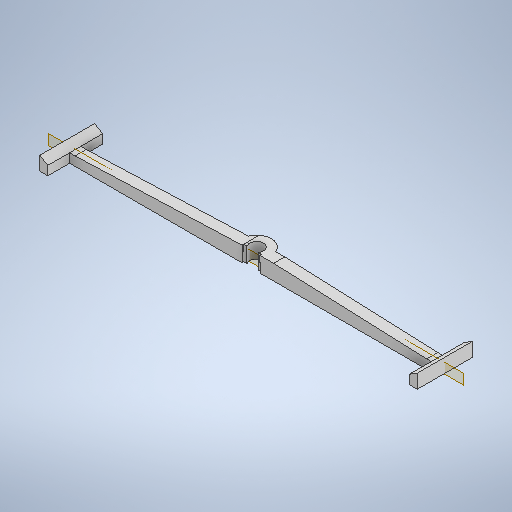
# Autodesk Inventor part: 2024_08_23_Holder_NMR_tube
Saved by Autodesk Inventor 2025.1 (Build 291241000, 241)
## iProperties
Created: 2024-08-23
Part Number: 2024_08_23_Holder_NMR_tube
Material: Generisch
Document SubType Name: Modeling
Designer: to86hug
Density: 1 g/cm^3
Appearance: Vorgabe
Author: to86hug
Autodesk Inventor part; units mm, degrees
ref_plane "YZ Plane" through (0, 0, 0) normal (1, 0, 0) x (0, 1, 0)
ref_plane "XZ Plane" through (0, 0, 0) normal (0, 1, 0) x (-1, 0, 0)
ref_plane "XY Plane" through (0, 0, 0) normal (0, 0, 1) x (1, 0, 0)
sketch "Skizze1" plane through (0, 0, 0) normal (0, 0, 1) x (1, 0, 0)
  line L0 (-68.016, 1.808) -> (67.584, 1.808)
  line L1 (67.584, 1.808) -> (67.584, -2.192)
  line L2 (67.584, -2.192) -> (-68.016, -2.192)
  line L3 (-68.016, -2.192) -> (-68.016, 1.808)
  line L4 (-68.016, 1.808) -> (67.584, -2.192) construction
  line L5 (67.584, 1.808) -> (-68.016, -2.192) construction
  point P0 (0, 0)
  point P1 (-0.216, -0.192)
  point P2 (-0.216, -0.192)
  dimension "d0" = 135.6
  dimension "d1" = 4
  constraints: 12 end point, 2 midpoint, 2 parallel, 1 horizontal, 1 perpendicular
  measures "d0" distance of L0.start L0.end
  measures "d1" distance of L0.end L1.end
extrude "Extrusion1" add sketch "Skizze1" along normal mid plane 3.25
ref_plane "Arbeitsebene1" through (-68.016, -0.192, 1.625) normal (0, -1, 0) x (1, 0, 0)
sketch "Skizze2" plane through (-68.016, -0.192, 1.625) normal (0, -1, 0) x (1, 0, 0)
  line L0 (0, -3.25) -> (0, 0) projected
  line L1 (0, -3.25) -> (135.6, -3.25) projected
  line L2 (0, 0) -> (2.85, 0)
  line L3 (2.85, 0) -> (2.85, -3.25)
  line L4 (2.85, -3.25) -> (0, -3.25)
  line L5 (0, -3.25) -> (0, 0)
  line L6 (0, 0) -> (0, 1.75)
  line L7 (0, 1.75) -> (2.85, 0)
  line L8 (135.6, -3.25) -> (135.6, 0) projected
  line L9 (135.6, 0) -> (132.75, 0)
  line L10 (132.75, 0) -> (132.75, -3.25)
  line L11 (132.75, -3.25) -> (135.6, -3.25)
  line L12 (135.6, -3.25) -> (135.6, 0)
  line L13 (135.6, 0) -> (135.6, 1.75)
  line L14 (135.6, 1.75) -> (132.75, 0)
  point P0 (68.016, -1.625)
  dimension "d4" = 2.85
  dimension "d5" = 1.75
  dimension "d6" = 2.85
  constraints: 24 end point, 4 parallel, 2 horizontal, 2 perpendicular, 2 point on line, 2 vertical
  measures "d4" distance of L3.end L4.end
  measures "d5" distance of L0.end L6.end
  measures "d6" distance of L11.end L10.end
extrude "Extrusion2" add sketch "Skizze2" along normal mid plane 19.7
sketch "Skizze3" plane through (0, 0, 1.625) normal (0, 0, 1) x (1, 0, 0)
  circle A0 centre (0, 0) radius 3.8975
  dimension "d9" = 7.795
  constraints: 1 centre point, 1 coincident
  measures "d9" diameter of A0
extrude "Extrusion3" cut sketch "Skizze3" against normal through all
sketch "Skizze4" plane through (0, 0, -1.625) normal (0, 0, -1) x (-1, 0, 0)
  line L0 (0.0769, -0.1614) -> (6.2269, -0.1614) construction
  circle A0 centre (0.0001, -0.1921) radius 2.495
  circle A1 centre (0.0001, -0.1921) radius 5.295
  line L1 (-24.5999, -1.5921) -> (24.6001, -1.5921)
  point P0 (-5.2949, -0.1921)
  point P1 (5.2951, -0.1921)
  point P2 (2.0653, -1.5921)
  point P3 (5.1066, -1.5921)
  point P4 (-5.1065, -1.5921)
  point P5 (-2.0651, -1.5921)
  dimension "d27" = 2.8
  dimension "d28" = 4.99
  dimension "d29" = 1.4
  constraints: 4 end point, 2 centre point, 2 coincident, 2 point on circle
  measures "d27" radial gap between concentric circles of A1 A0
  measures "d28" diameter of A0
  measures "d29" distance from line of A0.centre L1
extrude "Extrusion4" add sketch "Skizze4" against normal blind 5.5 contours A0 L1 A1 picked at (4.3097, 0.2335)
sketch "Skizze5" plane through (0, 0, 1.625) normal (0, 0, 1) x (1, 0, 0)
  line L0 (-4.9028, 1.808) -> (-65.166, 1.808) projected
  line L1 (-3.2227, -2.192) -> (-65.166, -2.192) projected
  line L2 (-3.2094, 1.808) -> (-63.2094, 1.808)
  line L3 (-63.2094, 1.808) -> (-63.2094, -2.192)
  line L4 (-63.2094, -2.192) -> (-3.2094, -2.192)
  line L5 (-3.2094, -2.192) -> (-3.2094, 1.808)
  line L6 (3.2227, -2.192) -> (64.734, -2.192) projected
  line L7 (3.1164, 1.808) -> (63.1164, 1.808)
  line L8 (63.1164, 1.808) -> (63.1164, -2.192)
  line L9 (63.1164, -2.192) -> (3.1164, -2.192)
  line L10 (3.1164, -2.192) -> (3.1164, 1.808)
  point P0 (0, 0)
  point P1 (-8.6889, 1.808)
  point P2 (-8.6001, -2.192)
  point P3 (8.6889, 1.808)
  point P4 (8.6001, -2.192)
  point P5 (3.1164, -2.192)
  point P6 (-3.2094, -2.192)
  point P7 (-63.2094, 1.808)
  point P8 (63.1164, -2.192)
  point P9 (-2.0688, 1.808)
  dimension "d17" = 60
  dimension "d18" = 60
  constraints: 16 end point, 4 parallel, 2 horizontal, 2 perpendicular
  measures "d17" distance of L4.end L3.end
  measures "d18" distance of L8.end L9.end
extrude "Extrusion5" add sketch "Skizze5" along normal blind 2.25
sketch "Skizze6" plane through (-65.166, -2.192, -1.625) normal (0, -1, 0) x (1, 0, 0)
  line L0 (1.9566, 5.5) -> (61.9566, 5.5) projected
  line L1 (1.9566, 5.5) -> (61.9566, 5.5)
  line L2 (56.9566, 5.5) -> (56.9566, 3.25)
  line L3 (56.9566, 3.25) -> (1.9566, 3.25)
  line L4 (1.9566, 3.25) -> (1.9566, 5.5)
  line L5 (61.9566, 5.5) -> (1.9566, 3.25)
  line L6 (128.2824, 3.25) -> (128.2824, 5.5) projected
  line L7 (128.2824, 5.5) -> (73.2824, 5.5)
  line L8 (73.2824, 5.5) -> (73.2824, 3.25)
  line L9 (73.2824, 3.25) -> (128.2824, 3.25)
  line L10 (128.2824, 3.25) -> (128.2824, 5.5)
  line L11 (73.2824, 5.5) -> (128.2824, 3.25)
  point P0 (65.166, 1.625)
  point P1 (56.5659, 5.5)
  point P2 (56.5659, 5.5)
  point P3 (56.5659, 5.5)
  dimension "d21" = 55
  dimension "d22" = 2.25
  dimension "d23" = 55
  dimension "d26" = 2.25
  constraints: 20 end point, 4 parallel, 2 horizontal, 2 perpendicular
  measures "d21" distance of L2.end L3.end
  measures "d22" vertical distance of L0.end L2.end
  measures "d23" distance of L9.end L8.end
  measures "d26" distance of L7.end L8.end
extrude "Extrusion6" cut sketch "Skizze6" against normal through all contours L0 L2 L5 L4 | L0 L5 L2 | L11 L7 L6
